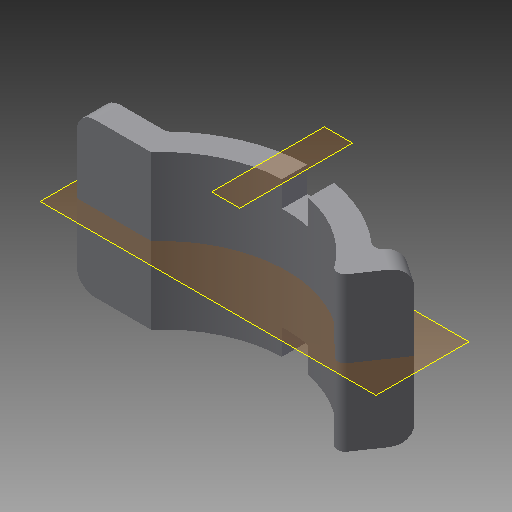
# Autodesk Inventor part: InteriorSw
Saved by Autodesk Inventor 2019 (Build 230136000, 136)
## iProperties
Created: 2016-05-14
Part Number: InteriorSw
Material: Genérico
Document SubType Name: Modeling
Designer: Isra
Density: 1 g/cm^3
Appearance: Valor por defecto
Author: Isra
Autodesk Inventor part; units mm, degrees
ref_plane "YZ Plane" through (0, 0, 0) normal (1, 0, 0) x (0, 1, 0)
ref_plane "XZ Plane" through (0, 0, 0) normal (0, 1, 0) x (-1, 0, 0)
ref_plane "XY Plane" through (0, 0, 0) normal (0, 0, 1) x (1, 0, 0)
sketch "Boceto1" plane through (0, 0, 0) normal (0, 1, 0) x (-1, 0, 0)
  arc A0 (0, 0) -> (4.0155, 1.6275) centre (-0.0005, 5.7684) ccw
  arc A1 (0, 0.9884) -> (3.6027, 2.6275) centre (-0.0005, 5.7684) ccw
  line L0 (4.0155, 1.6275) -> (5.0155, 1.6275)
  line L1 (6.0155, 1.6275) -> (6.5155, 1.6275)
  line L2 (6.5155, 1.6275) -> (6.5155, 2.6275)
  line L3 (6.5155, 2.6275) -> (3.6027, 2.6275)
  line L4 (0, 0.9884) -> (0, 0)
  arc A2 (-4.0155, 1.6275) -> (0, 0) centre (0.0005, 5.7684) ccw
  arc A3 (-4.0892, 3.294) -> (0, 0.9884) centre (0.0005, 5.7684) ccw
  line L5 (-4.0155, 1.6275) -> (-4.5782, 0.8009)
  line L6 (-4.5782, 0.8009) -> (-5.4045, 1.3641)
  line L7 (-5.4045, 1.3641) -> (-4.0892, 3.294)
  line L8 (5.0155, 1.6275) -> (6.0155, 1.6275)
  dimension "d1" = 4.78
  dimension "d2" = 1
  dimension "d3" = 1
  dimension "d4" = 0.5
  dimension "d5" = 1
  dimension "d6" = 1
  dimension "d7" = 1
  constraints: 18 end point, 10 point on circle, 4 centre point, 3 horizontal, 3 perpendicular, 3 symmetric about line, 2 coincident, 1 vertical, 2 other
  measures "d1" radius of A1
  measures "d2" distance of L0.start L0.end
  measures "d3" distance of L0.end L1.start
  measures "d4" distance of L1.start L1.end
  measures "d5" distance of L1.end L2.end
  measures "d6" distance of L5.start L5.end
  measures "d7" distance of L5.end L6.end
extrude "Extrusión1" add sketch "Boceto1" along normal mid plane 6
sketch "Boceto2" plane through (-4.0155, 3, 1.6275) normal (0, 0, -1) x (-1, 0, 0)
  line L0 (2.5, -6) -> (2.5, 0) projected
  line L1 (0, 0) -> (2.5, 0) projected
  line L2 (0, -6) -> (0, 0) projected
  line L3 (2.5, -6) -> (0, -6) projected
  circle A0 centre (1.25, -3) radius 0.8
  line L4 (1.25, -2.2) -> (1.25, -3.8)
  point P0 (-4.0155, -3)
  dimension "d10" = 1.6
  constraints: 2 end point, 2 point on circle, 1 centre point, 1 parallel
  measures "d10" diameter of A0
revolve "Revolución1" add sketch "Boceto2" angle 360 about axis through (-5.2655, 0.8, 1.6275) along (0, -1, 0) picked at (1.0732, -3.1996) contours L4 A0
ref_plane "Plano de trabajo1" through (0.9621, 4, -0.4105) normal (0, 1, 0) x (1, 0, 0)
sketch "Boceto3" plane through (0.9621, 4, -0.4105) normal (0, 1, 0) x (1, 0, 0)
  line L0 (0.027, -3.311) -> (-1.1061, -3.311)
  line L1 (-1.1061, -3.311) -> (-1.1061, 0.0355)
  line L2 (-1.1061, 0.0355) -> (0.027, 0.0355)
  line L3 (0.027, 0.0355) -> (0.027, -3.311)
  point P0 (-0.9621, -0.4105)
  dimension "d14" = 3.3465
  constraints: 8 end point, 2 parallel, 1 horizontal, 1 perpendicular
  measures "d14" distance between parallel lines of L2 L0
extrude "Extrusión2" cut sketch "Boceto3" against normal blind 2
ref_plane "Plano de trabajo2" through (0, 0, 0) normal (0, 1, 0) x (1, 0, 0)
mirror "Simetría1" about plane through (0, 0, 0) normal (0, 1, 0) of "Extrusión2"
fillet "Empalme1" radius 0.7 4 edges at (-6.5155, 3, 2.1275) (-6.5155, -3, 2.1275) (4.9914, -3, 1.0825) (4.9914, 3, 1.0825)
fillet "Empalme2" radius 0.3 1 edges at (4.0892, 0, 3.294)
fillet "Empalme3" radius 0.3 1 edges at (4.0155, 0, 1.6275)
